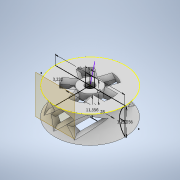
# Autodesk Inventor part: flyWheel2
Saved by Autodesk Inventor 2020 (Build 240168000, 168)
## iProperties
Created: 2020-08-21
Part Number: flyWheel2
Material: Generic
Document SubType Name: Modeling
Designer: buran
Density: 1 g/cm^3
Appearance: Default
Author: buran
Autodesk Inventor part; units mm, degrees
ref_plane "YZ Plane" through (0, 0, 0) normal (1, 0, 0) x (0, 1, 0)
ref_plane "XZ Plane" through (0, 0, 0) normal (0, 1, 0) x (-1, 0, 0)
ref_plane "XY Plane" through (0, 0, 0) normal (0, 0, 1) x (1, 0, 0)
sketch "Sketch1" plane through (0, 0, 0) normal (0, 0, 1) x (1, 0, 0)
  line L0 (-20, 7.7782) -> (20, 7.7782)
  line L1 (20, 7.7782) -> (20, -7.7782)
  line L2 (20, -7.7782) -> (-20, -7.7782)
  line L3 (-20, -7.7782) -> (-20, 7.7782)
  line L4 (-20, 0) -> (-16.778, 0)
  line L5 (20, 0) -> (16.778, 0)
  arc A0 (20, 7.7782) -> (20, -7.7782) centre (27.7776, 0) ccw
  arc A1 (-20, -7.7782) -> (-20, 7.7782) centre (-27.7776, 0) ccw
  line L6 (0, -7.7782) -> (0, 7.7782)
  line L7 (-14, 3.7778) -> (14, 3.7778)
  line L8 (14, 3.7778) -> (14, -7.7782)
  line L9 (14, -7.7782) -> (-14, -7.7782)
  line L10 (-14, -7.7782) -> (-14, 3.7778)
  line L11 (-2.5, 13) -> (2.5, 13)
  line L12 (2.5, 13) -> (2.5, 0)
  line L13 (2.5, 0) -> (-2.5, 0)
  line L14 (-2.5, 0) -> (-2.5, 13)
  line L15 (0, 0) -> (0, 13)
  point P0 (0, 0)
  point P1 (0, 3.7778)
  point P2 (-2.5, 3.7778)
  dimension "d0" = 15.5564
  dimension "d1" = 40
  dimension "d2" = 3.222
  dimension "d3" = 3.222
  dimension "d5" = 28
  dimension "d6" = 11.556
  dimension "d7" = 5
  dimension "d8" = 13
  constraints: 32 end point, 8 midpoint, 6 parallel, 6 point on circle, 5 horizontal, 4 perpendicular, 3 vertical alignment, 2 centre point, 2 horizontal alignment, 1 vertical
  measures "d0" distance of L0.end L1.end
  measures "d1" distance of L0.start L0.end
  measures "d2" distance of L4.start L4.end
  measures "d3" distance of L5.start L5.end
  measures "d5" distance between parallel lines of L8 L10
  measures "d6" distance between parallel lines of L9 L7
  measures "d7" distance of L11.start L11.end
  measures "d8" distance of L11.end L12.end
revolve "Revolution1" add sketch "Sketch1" angle 360 about axis through (0, -7.7782, 0) along (0, 1, 0) contours L0 L12 L7 L6 | L0 A0 L2 L8 L7 L12 | L7 L12 L13 L6 | L7 L8 L2 L6 L13 L12
revolve "Revolution2" cut sketch "Sketch1" angle 360 about axis through (0, 0, 0) along (0, 1, 0) contours L14 L11 L15 L0 | L0 L6 L7 L14 | L14 L13 L6 L2 L10 L7 | L7 L6 L13 L14
sketch "Sketch2" plane through (0, 7.7782, 0) normal (0, 1, 0) x (1, 0, 0)
  line L0 (0, 0) -> (-10.6222, 13.3083)
  line L1 (0, 0) -> (0, -20)
  circle A0 centre (0, 0) radius 20 projected
  constraints: 4 end point, 1 vertical, 1 vertical alignment, 1 other
ref_plane "Work Plane1" through (0, 7.7782, 20) normal (0, 0, 1) x (1, 0, 0)
sketch "Sketch3" plane through (0, 7.7782, 20) normal (0, 0, 1) x (1, 0, 0)
  line L0 (-20, -15.5563) -> (20, -15.5563) projected
  line L1 (0, -15.5563) -> (0, 0)
  line L2 (2.5, 0) -> (2.5, -4.0003) projected
  line L3 (-5.3033, -10.9602) -> (3.182, -2.4749)
  line L4 (3.182, -2.4749) -> (5.3033, -4.5962)
  line L5 (5.3033, -4.5962) -> (-3.182, -13.0815)
  line L6 (-3.182, -13.0815) -> (-5.3033, -10.9602)
  line L7 (-5.3033, -10.9602) -> (5.3033, -4.5962) construction
  line L8 (3.182, -2.4749) -> (-3.182, -13.0815) construction
  line L9 (-5.3033, -10.9602) -> (6.6967, -10.9602) construction
  line L10 (0, -7.7782) -> (2.1213, -7.7782)
  line L11 (15.3033, -4.5962) -> (6.818, -13.0815)
  line L12 (13.182, -2.4749) -> (15.3033, -4.5962)
  line L13 (4.6967, -10.9602) -> (13.182, -2.4749)
  line L14 (6.818, -13.0815) -> (4.6967, -10.9602)
  line L15 (-4.6967, -4.5962) -> (-13.182, -13.0815)
  line L16 (-6.818, -2.4749) -> (-4.6967, -4.5962)
  line L17 (-15.3033, -10.9602) -> (-6.818, -2.4749)
  line L18 (-13.182, -13.0815) -> (-15.3033, -10.9602)
  line L19 (5.3033, -4.5962) -> (-3.182, -13.0815)
  line L20 (3.182, -2.4749) -> (5.3033, -4.5962)
  line L21 (-5.3033, -10.9602) -> (3.182, -2.4749)
  line L22 (-3.182, -13.0815) -> (-5.3033, -10.9602)
  point P0 (12.1213, -7.7782)
  point P1 (-7.8787, -7.7782)
  dimension "d10" = 12
  dimension "d11" = 45
  dimension "d12" = 3
  dimension "d15" = 10
  dimension "d18" = 10
  constraints: 42 end point, 4 point on line, 3 horizontal, 3 midpoint, 3 parallel, 2 perpendicular, 1 equal length, 27 other
  measures "d10" distance of L3.start L3.end
  measures "d11" angle of L9 L3
  measures "d12" distance of L3.end L4.end
  measures "d15" distance of L4.end L11.start
  measures "d18" distance of L4.end L15.start
extrude "Extrusion1" cut sketch "Sketch3" against normal through all
chamfer "Chamfer1" distance 2 angle 45 12 edges at (-11.1644, 0.9569, -12.5801) (-11.1644, 0.9569, 12.5801) (-8.8831, -1.0045, -14.2876) (-8.8831, -1.0045, 14.2876) (-1.0305, 1.0908, -16.8006) (-1.0305, 1.0908, 16.8006) (1.0306, -1.0907, -16.8006) (1.0306, -1.0907, 16.8006) (8.8831, 1.0044, -14.2876) (8.8831, 1.0044, 14.2876) (11.1644, -0.957, -12.5801) (11.1644, -0.957, 12.5801)
sketch "Sketch4" plane through (0, 7.7782, 0) normal (0, 1, 0) x (1, 0, 0)
  circle A0 centre (0, 0) radius 6
  circle A1 centre (0, 0) radius 12.5
  line L0 (12.369, 1.8051) -> (5.722, 1.8051)
  line L1 (5.722, -1.8051) -> (12.369, -1.8051)
  line L2 (2.1055, 12.3214) -> (0.0515, 5.9998)
  line L3 (3.4849, 4.8842) -> (5.5389, 11.2058)
  line L4 (-11.0677, 5.81) -> (-5.6902, 1.903)
  line L5 (-3.5682, 4.8236) -> (-8.9457, 8.7306)
  line L6 (-8.9457, -8.7306) -> (-3.5682, -4.8236)
  line L7 (-5.6902, -1.903) -> (-11.0677, -5.81)
  line L8 (5.5389, -11.2058) -> (3.4849, -4.8842)
  line L9 (0.0515, -5.9998) -> (2.1055, -12.3214)
  point P0 (7.3231, 0)
  point P1 (2.263, 6.9647)
  point P2 (-5.9245, 4.3044)
  point P3 (-5.9245, -4.3044)
  point P4 (2.263, -6.9647)
  point P5 (3.4849, 4.8842)
  point P6 (5.5389, 11.2058)
  point P7 (2.1055, 12.3214)
  point P8 (0.0515, 5.9998)
  point P9 (-3.5682, 4.8236)
  point P10 (-11.0677, 5.81)
  point P11 (-5.6902, 1.903)
  point P12 (-5.6902, -1.903)
  point P13 (-11.0677, -5.81)
  point P14 (-8.9457, -8.7306)
  point P15 (-3.5682, -4.8236)
  point P16 (0.0515, -5.9998)
  point P17 (2.1055, -12.3214)
  point P18 (5.5389, -11.2058)
  point P19 (3.4849, -4.8842)
  dimension "d26" = 12
  dimension "d27" = 25
  dimension "d30" = 360
  constraints: 20 end point, 4 point on circle, 2 centre point, 2 coincident, 1 horizontal, 1 parallel, 36 other
  measures "d26" diameter of A0
  measures "d27" diameter of A1
extrude "Extrusion2" cut sketch "Sketch4" against normal blind 10 contours A0 L0 A1 L1 | A0 L2 A1 L3 | L8 A1 L9 A0 | A0 L4 A1 L5 | L6 A1 L7 A0
chamfer "Chamfer2" distance 2 angle 45 10 edges at (-8.379, 7.7782, 3.8565) (-6.257, 7.7782, 6.7771) (1.0785, 7.7782, 9.1606) (4.5119, 7.7782, 8.045) (9.0455, 7.7782, 1.8051) (9.0455, 7.7782, -1.8051) (4.5119, 7.7782, -8.045) (1.0785, 7.7782, -9.1606) (-6.257, 7.7782, -6.7771) (-8.379, 7.7782, -3.8565)
body "Solid1"
